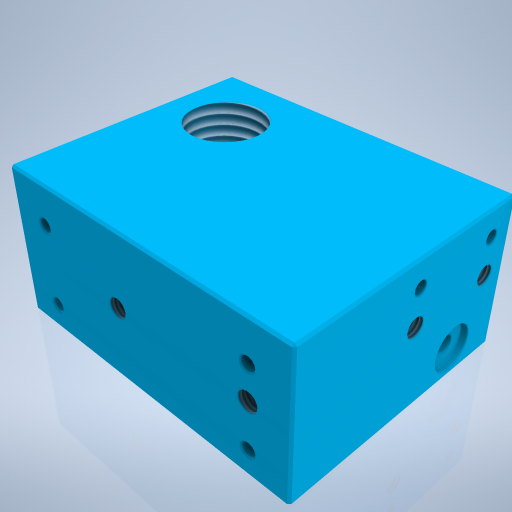
# Autodesk Inventor part: Steuerblock
Saved by Autodesk Inventor 2024.2 (Build 282272000, 272)
## iProperties
Created: 2024-04-22
Part Number: Steuerblock
Material: Stahl, Legierung
Document SubType Name: Modeling
Designer: Fabri
Density: 7.73 g/cm^3
Appearance: Himmelblau - mittel
Author: Fabri
Autodesk Inventor part; units mm, degrees
ref_plane "XZ Plane" through (0, 0, 0) normal (0, 1, 0) x (-1, 0, 0)
ref_plane "XY Plane" through (0, 0, 0) normal (0, 0, 1) x (1, 0, 0)
sketch "Skizze1" plane through (0, 0, 0) normal (0, 0, 1) x (1, 0, 0)
  line L0 (-34.75, -27.5) -> (34.75, -27.5)
  line L1 (34.75, -27.5) -> (34.75, 27.5)
  line L2 (34.75, 27.5) -> (-34.75, 27.5)
  line L3 (-34.75, 27.5) -> (-34.75, -27.5)
  line L4 (-34.75, -27.5) -> (34.75, 27.5) construction
  line L5 (34.75, -27.5) -> (-34.75, 27.5) construction
  point P0 (0, 0)
  dimension "d0" = 69.5
  dimension "d1" = 55
  constraints: 12 end point, 2 midpoint, 2 parallel, 1 horizontal, 1 perpendicular
  measures "d0" distance between parallel lines of L1 L3
  measures "d1" distance between parallel lines of L0 L2
extrude "Extrusion1" add sketch "Skizze1" against normal blind 33
sketch "Skizze2" plane through (0, 0, 0) normal (0, 0, 1) x (1, 0, 0)
  line L0 (-34.75, 27.5) -> (-34.75, -27.5) projected
  line L1 (-34.75, -27.5) -> (34.75, -27.5) projected
  point P0 (0, 0)
  point P1 (-19.75, 11.5)
  dimension "d11" = 15
  dimension "d12" = 39
  measures "d11" distance from line of point (-19.75, 11.5) L0
  measures "d12" distance from line of L1 point (-19.75, 11.5)
hole "Bohrung1" at (-19.75, 11.5, 0) direction (0, 0, -1) diameter 17.294 depth 23 tip angle 118 thread size "M20x2.5" class "6H" standard "ISO Metric profile"
sketch "Skizze4" plane through (34.75, -27.5, 0) normal (1, 0, 0) x (0, 0, -1)
  line L0 (0, 0) -> (33, 0) projected
  line L1 (33, 55) -> (33, 0) projected
  point P0 (0, 27.5)
  point P1 (6, 49)
  point P2 (14, 49)
  point P3 (6, 29)
  point P4 (14, 29)
  dimension "d21" = 29
  dimension "d22" = 20
  dimension "d23" = 27
  dimension "d24" = 27
  dimension "d85" = 8
  constraints: 2 horizontal alignment, 1 vertical alignment
  measures "d21" distance from line of L0 point (6, 29)
  measures "d22" distance of point (6, 29) point (6, 49)
  measures "d23" distance from line of L1 point (6, 49)
  measures "d24" distance from line of L1 point (6, 29)
  measures "d85" distance of point (14, 49) point (6, 49)
hole "Bohrung3" at (34.75, 21.5, -14) at (34.75, 1.5, -14) direction (-1, 0, 0) diameter 4.134 depth 15 tip angle 118 thread size "M5x0.8" class "6H" standard "ISO Metric profile"
hole "Bohrung4" at (34.75, 21.5, -6) at (34.75, 1.5, -6) direction (-1, 0, 0) diameter 3 depth 8 tip angle 118
sketch "Skizze5" plane through (34.75, -27.5, 0) normal (1, 0, 0) x (0, 0, -1)
  line L0 (33, 55) -> (33, 0) projected
  line L1 (0, 0) -> (0, 55) projected
  line L2 (0, 42) -> (33, 42) construction
  line L3 (0, 55) -> (33, 55) projected
  point P0 (0, 27.5)
  point P1 (26.5, 42)
  point P2 (16.5, 42)
  dimension "d48" = 6.5
  dimension "d49" = 13
  constraints: 2 end point, 2 point on line, 1 horizontal alignment, 1 midpoint, 1 perpendicular
  measures "d48" distance from line of L0 point (26.5, 42)
  measures "d49" distance from line of point (16.5, 42) L3
hole "Bohrung5" at (34.75, 14.5, -26.5) direction (-1, 0, 0) diameter 4 depth 50 counterbore diameter 10 counterbore depth 1.5
sketch "Skizze6" plane through (-34.75, -27.5, 0) normal (0, -1, 0) x (1, 0, 0)
  line L0 (69.5, -33) -> (0, -33) projected
  line L1 (69.5, 0) -> (69.5, -33) projected
  line L2 (69.5, -16.5) -> (0, -16.5) construction
  point P0 (34.75, 0)
  point P1 (60.5, -27)
  point P2 (60.5, -9)
  dimension "d57" = 6
  dimension "d58" = 18
  dimension "d59" = 9
  dimension "d60" = 9
  constraints: 2 end point, 1 horizontal, 1 midpoint
  measures "d57" distance from line of L0 point (60.5, -27)
  measures "d58" distance of point (60.5, -27) point (60.5, -9)
  measures "d59" distance from line of L1 point (60.5, -27)
  measures "d60" distance from line of L1 point (60.5, -9)
hole "Bohrung6" at (25.75, -27.5, -27) at (25.75, -27.5, -9) direction (0, 1, 0) diameter 3.2 depth 8 tip angle 118
sketch "Skizze7" plane through (-34.75, -27.5, 0) normal (0, -1, 0) x (1, 0, 0)
  circle A0 centre (60.5, -27) radius 1.6 projected
  line L0 (69.5, 0) -> (69.5, -33) projected
  point P0 (34.75, 0)
  point P1 (60.5, -16.5)
  point P2 (69.5, -16.5)
  constraints: 1 horizontal alignment, 1 midpoint, 1 vertical alignment
hole "Bohrung7" at (25.75, -27.5, -16.5) direction (0, 1, 0) diameter 4.134 depth 17 tip angle 118 thread size "M5x0.8" class "6H" standard "ISO Metric profile"
ref_plane "Arbeitsebene1" through (0, 0, 0) normal (1, 0, 0) x (0, 1, 0)
mirror "Spiegeln1" about plane through (0, 0, 0) normal (1, 0, 0) of "Bohrung6"
sketch "Skizze8" plane through (-34.75, -27.5, 0) normal (0, -1, 0) x (1, 0, 0)
  line L0 (69.5, 0) -> (69.5, -33) projected
  line L1 (0, 0) -> (0, -33) projected
  line L2 (69.5, 0) -> (69.5, -33) projected
  line L3 (0, 0) -> (69.5, 0) projected
  point P0 (34.75, 0)
  point P1 (29, -16.5)
  point P2 (69.5, -16.5)
  point P3 (69.5, -16.5)
  dimension "d76" = 29
  dimension "d77" = 16.5
  constraints: 2 horizontal alignment, 2 midpoint
  measures "d76" distance from line of L1 point (29, -16.5)
  measures "d77" distance from line of L3 point (29, -16.5)
hole "Bohrung8" at (-5.75, -27.5, -16.5) direction (0, 1, 0) diameter 4.134 depth 17 tip angle 118 thread size "M5x0.8" class "6H" standard "ISO Metric profile"
chamfer "Fasen1" distance 0.5 angle 45 11 edges at (34.75, 0, 0) (0, 27.5, 0) (-34.75, 0, 0) (0, -27.5, 0) (34.75, -27.5, -16.5) (34.75, 0, -33) (34.75, 27.5, -16.5) (-34.75, 27.5, -16.5) (0, 27.5, -33) (0, -27.5, -33) (-34.75, -27.5, -16.5)
chamfer "Fasen2" distance 0.5 angle 45 1 edges at (-34.75, 0, -33)
equation "\"d24\" = d23"
equation "\"d60\" = d59"
